Autodesk Inventor part; units mm, degrees
(part 4 of 4)
sketch "Sketch10" plane through (0, 0, 0) normal (0, 1, 0) x (1, 0, 0)
  circle A0 centre (29.25, 48.75) radius 2.8 construction
  circle A1 centre (29.25, 29.25) radius 2.8 construction
  circle A2 centre (29.25, 9.75) radius 2.8 construction
  circle A3 centre (29.25, -9.75) radius 2.8 construction
  circle A4 centre (29.25, -29.25) radius 2.8 construction
  circle A5 centre (29.25, -48.75) radius 2.8 construction
  circle A6 centre (9.75, 48.75) radius 2.8 construction
  circle A7 centre (-9.75, 48.75) radius 2.8 construction
  circle A8 centre (-29.25, 48.75) radius 2.8 construction
  circle A9 centre (29.25, 48.75) radius 2.8
  circle A10 centre (29.25, 29.25) radius 2.8
  circle A11 centre (29.25, 9.75) radius 2.8
  circle A12 centre (29.25, -9.75) radius 2.8
  circle A13 centre (29.25, -29.25) radius 2.8
  circle A14 centre (29.25, -48.75) radius 2.8
  circle A15 centre (9.75, 48.75) radius 2.8
  circle A16 centre (9.75, 29.25) radius 2.8
  circle A17 centre (9.75, 9.75) radius 2.8
  circle A18 centre (9.75, -9.75) radius 2.8
  circle A19 centre (9.75, -29.25) radius 2.8
  circle A20 centre (9.75, -48.75) radius 2.8
  circle A21 centre (-9.75, 48.75) radius 2.8
  circle A22 centre (-9.75, 29.25) radius 2.8
  circle A23 centre (-9.75, 9.75) radius 2.8
  circle A24 centre (-9.75, -9.75) radius 2.8
  circle A25 centre (-9.75, -29.25) radius 2.8
  circle A26 centre (-9.75, -48.75) radius 2.8
  circle A27 centre (-29.25, 48.75) radius 2.8
  circle A28 centre (-29.25, 29.25) radius 2.8
  circle A29 centre (-29.25, 9.75) radius 2.8
  circle A30 centre (-29.25, -9.75) radius 2.8
  circle A31 centre (-29.25, -29.25) radius 2.8
  circle A32 centre (-29.25, -48.75) radius 2.8
  point P0 (0, 0)
  dimension "d378" = 5.6
  dimension "d379" = 5.6
  dimension "d380" = 5.6
  dimension "d381" = 5.6
  dimension "d382" = 5.6
  dimension "d383" = 5.6
  dimension "d384" = 5.6
  dimension "d385" = 5.6
  dimension "d386" = 5.6
  dimension "d387" = 5.6
  dimension "d388" = 5.6
  dimension "d389" = 5.6
  dimension "d390" = 5.6
  dimension "d391" = 5.6
  dimension "d392" = 5.6
  dimension "d393" = 5.6
  dimension "d394" = 5.6
  dimension "d395" = 5.6
  dimension "d396" = 5.6
  dimension "d397" = 5.6
  dimension "d398" = 5.6
  dimension "d399" = 5.6
  dimension "d400" = 5.6
  dimension "d401" = 5.6
  constraints: 24 centre point, 6 coincident
  measures "d378" diameter of A9
  measures "d379" diameter of A10
  measures "d380" diameter of A11
  measures "d381" diameter of A12
  measures "d382" diameter of A13
  measures "d383" diameter of A14
  measures "d384" diameter of A15
  measures "d385" diameter of A16
  measures "d386" diameter of A17
  measures "d387" diameter of A18
  measures "d388" diameter of A19
  measures "d389" diameter of A20
  measures "d390" diameter of A21
  measures "d391" diameter of A22
  measures "d392" diameter of A23
  measures "d393" diameter of A24
  measures "d394" diameter of A25
  measures "d395" diameter of A26
  measures "d396" diameter of A27
  measures "d397" diameter of A28
  measures "d398" diameter of A29
  measures "d399" diameter of A30
  measures "d400" diameter of A31
  measures "d401" diameter of A32
sketch "Sketch11" plane through (0, 0, 0) normal (0, 1, 0) x (1, 0, 0)
  circle A0 centre (17.1945, 60.0191) radius 0.75 projected
  circle A1 centre (9.6945, 60.0191) radius 0.75 projected
  circle A2 centre (-2.3055, 60.0191) radius 0.75 projected
  circle A3 centre (-21.8055, 60.0191) radius 0.75 projected
  circle A4 centre (-29.3055, 60.0191) radius 0.75 projected
  circle A5 centre (29.3055, -60.0191) radius 0.75 projected
  circle A6 centre (21.8055, -60.0191) radius 0.75 projected
  circle A7 centre (9.8055, -60.0191) radius 0.75 projected
  circle A8 centre (2.3055, -60.0191) radius 0.75 projected
  circle A9 centre (-9.6945, -60.0191) radius 0.75 projected
  circle A10 centre (-17.1945, -60.0191) radius 0.75 projected
  line L0 (17.1945, 60.0191) -> (9.6945, 60.0191) construction
  circle A11 centre (-9.8055, 60.0191) radius 0.75 projected
  line L1 (-9.8055, 60.0191) -> (-2.3055, 60.0191) construction
  line L2 (-21.8055, 60.0191) -> (-29.3055, 60.0191) construction
  line L3 (-17.1945, -60.0191) -> (-9.6945, -60.0191) construction
  line L4 (2.3055, -60.0191) -> (9.8055, -60.0191) construction
  line L5 (29.3055, -60.0191) -> (21.8055, -60.0191) construction
  circle A12 centre (29.25, -48.75) radius 2.8 projected
  circle A13 centre (-29.25, 48.75) radius 2.8 projected
  line L6 (-29.25, 48.75) -> (-43.25, 48.75) construction
  line L7 (29.25, -48.75) -> (43.25, -48.75) construction
  circle A14 centre (43.25, -48.75) radius 1.25
  circle A15 centre (25.5555, -60.0191) radius 1.25
  circle A16 centre (6.0555, -60.0191) radius 1.25
  circle A17 centre (-13.4445, -60.0191) radius 1.25
  circle A18 centre (-25.5555, 60.0191) radius 1.25
  circle A19 centre (-6.0555, 60.0191) radius 1.25
  circle A20 centre (13.4445, 60.0191) radius 1.25
  circle A21 centre (-43.25, 48.75) radius 1.25
  point P0 (0, 0)
  dimension "d526" = 14
  dimension "d527" = 14
  dimension "d528" = 2.5
  dimension "d529" = 2.5
  dimension "d530" = 2.5
  dimension "d532" = 2.5
  dimension "d533" = 2.5
  dimension "d534" = 2.5
  dimension "d535" = 2.5
  dimension "d536" = 2.5
  constraints: 16 end point, 8 centre point, 8 horizontal, 6 midpoint, 2 coincident
  measures "d526" distance of L6.start L6.end
  measures "d527" distance of L7.start L7.end
  measures "d528" diameter of A14
  measures "d529" diameter of A15
  measures "d530" diameter of A16
  measures "d532" diameter of A17
  measures "d533" diameter of A18
  measures "d534" diameter of A19
  measures "d535" diameter of A20
  measures "d536" diameter of A21
extrude "Extrusion3" add sketch "Sketch7" along normal blind 6 contours A6 L10 L11 L9 | L9 L11 L10 A6 | L16 L15 A8 L14 | L14 A8 L15 L16 | A7 L29 L28 L27 | L27 L28 L29 A7 | L42 L41 A9 L40 | L40 A9 L41 L42 | L51 L50 A10 L49 | L49 A10 L50 L51 | A11 L155 L157 L156 | L156 L157 L155 A11 | A53 L185 L184 L183 | L183 L184 L185 A53 | L203 A54 L200 L189 | L189 L200 A54 L203 | L198 A55 L199 L190 | L190 L199 A55 L198 | L206 A56 L209 L191 | L191 L209 A56 L206 | A59 L204 L195 L192 | L192 L195 L204 A59 | L211 A60 L210 L205 | L205 L210 A60 L211 | A105 L335 L334 L333 | L333 L334 L335 A105 | L353 A106 L350 L339 | L339 L350 A106 L353 | L348 A107 L349 L340 | L340 L349 A107 L348 | L356 A108 L359 L341 | L341 L359 A108 L356 | A111 L354 L345 L342 | L342 L345 L354 A111 | L361 A112 L360 L355 | L355 L360 A112 L361 | A151 L485 L484 L483 | L483 L484 L485 A151 | L503 A152 L500 L489 | L489 L500 A152 L503 | L498 A153 L499 L490 | L490 L499 A153 L498 | L506 A154 L509 L491 | L491 L509 A154 L506 | A157 L504 L495 L492 | L492 L495 L504 A157 | L511 A158 L510 L505 | L505 L510 A158 L511 | A197 L635 L634 L633 | L633 L634 L635 A197 | L653 A198 L650 L639 | L639 L650 A198 L653 | L648 A199 L649 L640 | L640 L649 A199 L648 | L656 A200 L659 L641 | L641 L659 A200 L656 | A203 L654 L645 L642 | L642 L645 L654 A203 | L661 A204 L660 L655 | L655 L660 A204 L661 | L913 L917 L912 A269 | A269 L912 L917 L913 | A286 L780 L920 L779 | L779 L920 L780 A286 | A287 L784 L921 L787 | L787 L921 L784 A287 | A288 L791 L922 L792 | L792 L922 L791 A288 | L916 L796 A278 L795 | L795 A278 L796 L916 | L800 L803 A243 L799 | L799 A243 L803 L800 | L1063 L1067 L1062 A315 | A315 L1062 L1067 L1063 | A332 L930 L1070 L929 | L929 L1070 L930 A332 | A333 L934 L1071 L937 | L937 L1071 L934 A333 | A334 L941 L1072 L942 | L942 L1072 L941 A334 | L1066 L946 A324 L945 | L945 A324 L946 L1066 | L950 L953 A289 L949 | L949 A289 L953 L950 | L1213 L1217 L1212 A361 | A361 L1212 L1217 L1213 | A378 L1080 L1220 L1079 | L1079 L1220 L1080 A378 | A379 L1084 L1221 L1087 | L1087 L1221 L1084 A379 | A380 L1091 L1222 L1092 | L1092 L1222 L1091 A380 | L1216 L1096 A370 L1095 | L1095 A370 L1096 L1216 | L1100 L1103 A335 L1099 | L1099 A335 L1103 L1100
extrude "Extrusion4" add sketch "Sketch7" along normal blind 0.5 contours L3 A33 L65 A35 L76 L172 L77 A34 L67 A32 L4 A22 L6 A31 L10 A6 L9 A30 L5 A23 | A6 L10 L11 L9 | L14 A8 L15 L16 | L14 A29 L19 A20 L32 A37 L81 A45 L84 L118 L117 L173 L119 A44 L83 A36 L33 A21 L20 A28 L15 A8 | A45 L118 L84 | A19 L36 A39 L99 A47 L101 L123 L122 L174 L124 A46 L100 A38 L37 A18 L24 A27 L29 A7 L27 A26 L23 | A7 L29 L28 L27 | A47 L123 L101 | L40 A9 L41 L42 | L40 A25 L45 A17 L60 A41 L90 A49 L92 L115 L175 L127 A48 L91 A40 L61 A16 L46 A24 L41 A9 | A49 L126 L92 | L126 A49 L125 L175 L115 | L51 L50 A10 L49 | A10 L50 A13 L54 A14 L56 A43 L95 A50 L130 L176 L131 A51 L96 A42 L57 A15 L55 A12 L49 | L156 L157 L155 A11 | A11 L155 L177 L156 | L183 A53 L185 L188 | L183 L184 L185 A53 | L189 L200 A54 L203 | A54 L200 A63 L215 A68 L278 A93 L308 A96 L319 L321 L316 A95 L311 A94 L277 A65 L216 A64 L203 | L198 A55 L199 L190 | L198 A69 L218 A78 L286 A86 L264 A85 L263 L268 L270 L272 L269 A88 L266 A87 L283 A77 L221 A70 L199 A55 | A85 L268 L263 | L206 A56 L209 L191 | L206 A75 L231 A73 L232 A79 L239 A82 L245 L247 L240 A81 L237 A80 L233 A72 L228 A74 L209 A56 | A57 L223 A66 L282 A89 L296 A92 L291 L301 L299 L297 L298 A91 L292 A90 L279 A67 L224 A58 L204 A59 L192 | A59 L204 L195 L192 | A92 L301 L291 | L205 L210 A60 L211 | A60 L210 A62 L229 A76 L288 A97 L324 A84 L262 L258 L253 L256 A83 L327 A98 L287 A71 L226 A61 L211 | A84 L261 L262 | L261 A84 L257 L253 L258 | L333 A105 L335 L338 | L333 L334 L335 A105 | L339 L350 A106 L353 | A106 L350 A115 L365 A120 L428 A145 L458 A148 L469 L471 L466 A147 L461 A146 L427 A117 L366 A116 L353 | L348 A107 L349 L340 | L348 A121 L368 A130 L436 A138 L414 A137 L413 L418 L420 L422 L419 A140 L416 A139 L433 A129 L371 A122 L349 A107 | A137 L418 L413 | L356 A108 L359 L341 | L356 A127 L381 A125 L382 A131 L389 A134 L395 L397 L390 A133 L387 A132 L383 A124 L378 A126 L359 A108 | A109 L373 A118 L432 A141 L446 A144 L441 L451 L449 L447 L448 A143 L442 A142 L429 A119 L374 A110 L354 A111 L342 | A111 L354 L345 L342 | A144 L451 L441 | L355 L360 A112 L361 | A112 L360 A114 L379 A128 L438 A149 L474 A136 L412 L408 L403 L406 A135 L477 A150 L437 A123 L376 A113 L361 | A136 L411 L412 | L411 A136 L407 L403 L408 | L483 A151 L485 L488 | L483 L484 L485 A151 | L489 L500 A152 L503 | A152 L500 A161 L515 A166 L578 A191 L608 A194 L619 L621 L616 A193 L611 A192 L577 A163 L516 A162 L503 | L498 A153 L499 L490 | L498 A167 L518 A176 L586 A184 L564 A183 L563 L568 L570 L572 L569 A186 L566 A185 L583 A175 L521 A168 L499 A153 | A183 L568 L563 | L506 A154 L509 L491 | L506 A173 L531 A171 L532 A177 L539 A180 L545 L547 L540 A179 L537 A178 L533 A170 L528 A172 L509 A154 | A155 L523 A164 L582 A187 L596 A190 L591 L601 L599 L597 L598 A189 L592 A188 L579 A165 L524 A156 L504 A157 L492 | A157 L504 L495 L492 | A190 L601 L591 | L505 L510 A158 L511 | A158 L510 A160 L529 A174 L588 A195 L624 A182 L562 L558 L553 L556 A181 L627 A196 L587 A169 L526 A159 L511 | A182 L561 L562 | L561 A182 L557 L553 L558 | L633 A197 L635 L638 | L633 L634 L635 A197 | L639 L650 A198 L653 | A198 L650 A207 L665 A212 L728 A237 L758 A240 L769 L771 L766 A239 L761 A238 L727 A209 L666 A208 L653 | L648 A199 L649 L640 | L648 A213 L668 A222 L736 A230 L714 A229 L713 L718 L720 L722 L719 A232 L716 A231 L733 A221 L671 A214 L649 A199 | A229 L718 L713 | L656 A200 L659 L641 | L656 A219 L681 A217 L682 A223 L689 A226 L695 L697 L690 A225 L687 A224 L683 A216 L678 A218 L659 A200 | A201 L673 A210 L732 A233 L746 A236 L741 L751 L749 L747 L748 A235 L742 A234 L729 A211 L674 A202 L654 A203 L642 | A203 L654 L645 L642 | A236 L751 L741 | L655 L660 A204 L661 | A204 L660 A206 L679 A220 L738 A241 L774 A228 L712 L708 L703 L706 A227 L777 A242 L737 A215 L676 A205 L661 | A228 L711 L712 | L711 A228 L707 L703 L708 | L778 A276 L813 A261 L898 A268 L900 L908 L905 L903 L904 A267 L899 A262 L814 A277 L821 A273 L912 A269 L913 A272 | A269 L912 L917 L913 | A268 L908 L900 | L779 A286 L780 A283 L789 A245 L836 A254 L846 A255 L845 L851 L854 L859 A256 L849 A253 L837 A279 L918 A280 | L779 L920 L780 A286 | L851 L850 A255 L858 L854 | A255 L850 L845 | A281 L809 A258 L862 A259 L864 L867 L872 L871 L870 A260 L863 A257 L812 A282 L806 A271 L784 A287 L787 A270 L783 | A287 L784 L921 L787 | A259 L867 L864 | A248 L822 A249 L826 A251 L834 L833 L830 A252 L828 A250 L823 A246 L835 A244 L791 A288 L792 A247 L790 | A288 L791 L922 L792 | L795 A278 L796 L916 | L795 A285 L808 A275 L816 A264 L877 A266 L889 L894 L888 A265 L879 A263 L817 A274 L909 A284 L796 A278 | L799 A243 L803 L800 | L799 L802 L803 A243 | L928 A322 L963 A307 L1048 A314 L1050 L1058 L1055 L1053 L1054 A313 L1049 A308 L964 A323 L971 A319 L1062 A315 L1063 A318 | A315 L1062 L1067 L1063 | A314 L1058 L1050 | L929 A332 L930 A329 L939 A291 L986 A300 L996 A301 L995 L1001 L1004 L1009 A302 L999 A299 L987 A325 L1068 A326 | L929 L1070 L930 A332 | L1001 L1000 A301 L1008 L1004 | A301 L1000 L995 | A327 L959 A304 L1012 A305 L1014 L1017 L1022 L1021 L1020 A306 L1013 A303 L962 A328 L956 A317 L934 A333 L937 A316 L933 | A333 L934 L1071 L937 | A305 L1017 L1014 | A294 L972 A295 L976 A297 L984 L983 L980 A298 L978 A296 L973 A292 L985 A290 L941 A334 L942 A293 L940 | A334 L941 L1072 L942 | L945 A324 L946 L1066 | L945 A331 L958 A321 L966 A310 L1027 A312 L1039 L1044 L1038 A311 L1029 A309 L967 A320 L1059 A330 L946 A324 | L949 A289 L953 L950 | L949 L952 L953 A289 | L1078 A368 L1113 A353 L1198 A360 L1200 L1208 L1205 L1203 L1204 A359 L1199 A354 L1114 A369 L1121 A365 L1212 A361 L1213 A364 | A361 L1212 L1217 L1213 | A360 L1208 L1200 | L1079 A378 L1080 A375 L1089 A337 L1136 A346 L1146 A347 L1145 L1151 L1154 L1159 A348 L1149 A345 L1137 A371 L1218 A372 | L1079 L1220 L1080 A378 | L1151 L1150 A347 L1158 L1154 | A347 L1150 L1145 | A373 L1109 A350 L1162 A351 L1164 L1167 L1172 L1171 L1170 A352 L1163 A349 L1112 A374 L1106 A363 L1084 A379 L1087 A362 L1083 | A379 L1084 L1221 L1087 | A351 L1167 L1164 | A340 L1122 A341 L1126 A343 L1134 L1133 L1130 A344 L1128 A342 L1123 A338 L1135 A336 L1091 A380 L1092 A339 L1090 | A380 L1091 L1222 L1092 | L1095 A370 L1096 L1216 | L1095 A377 L1108 A367 L1116 A356 L1177 A358 L1189 L1194 L1188 A357 L1179 A355 L1117 A366 L1209 A376 L1096 A370 | L1099 A335 L1103 L1100 | L1099 L1102 L1103 A335 picked at (41.2772, -59.7704) picked at (39.0702, -55.2707) picked at (37.2772, -59.7707) picked at (35.0702, -55.2707) picked at (33.2772, -59.7707) picked at (29.3405, -59.7709) picked at (29.1595, 59.7709) picked at (17.1662, 59.7704) picked at (21.2228, 59.7707) picked at (25.2228, 59.7707) picked at (19.4864, 55.2707) picked at (23.4864, 55.2707) picked at (9.6595, 59.7709) picked at (-2.3338, 59.7704) picked at (1.7228, 59.7707) picked at (5.7228, 59.7707) picked at (-0.0136, 55.2707) picked at (3.9864, 55.2707) picked at (-9.8405, 59.7709) picked at (-21.8338, 59.7704) picked at (-17.7772, 59.7707) picked at (-13.8338, 59.7707) picked at (-19.5136, 55.2707) picked at (-15.5702, 55.2707) picked at (-29.3405, 59.7709) picked at (-41.3338, 59.7704) picked at (-37.3338, 59.7707) picked at (-33.3338, 59.7707) picked at (-39.0702, 55.2707) picked at (-35.0702, 55.2707) picked at (19.5702, -55.2707) picked at (15.5702, -55.2707) picked at (17.8338, -59.7707) picked at (13.8338, -59.7707) picked at (21.7772, -59.7704) picked at (9.8405, -59.7709) picked at (0.0702, -55.2707) picked at (-3.9298, -55.2707) picked at (-1.6662, -59.7707) picked at (-5.6662, -59.7707) picked at (2.2772, -59.7704) picked at (-9.6595, -59.7709) picked at (-19.4298, -55.2707) picked at (-23.4298, -55.2707) picked at (-21.1662, -59.7707) picked at (-25.1662, -59.7707) picked at (-17.2228, -59.7704) picked at (-29.1595, -59.7709)
extrude "Extrusion5" add sketch "Sketch10" along normal blind 6
extrude "Extrusion6" add sketch "Sketch7" along normal blind 4 contours L163 L74 L75 L73 L162 L172 | L164 L135 L134 L136 L165 L173 | L166 L139 L138 L140 L167 L174 | L175 L168 L142 L141 L143 L169 | L176 L147 L145 L144 L146 L148 | L177 L160 L153 L152 L154 L161 | L179 L188 L181 L182 L180 L178 | L322 L315 L314 L318 L317 L321 | L272 L273 L276 L275 L274 L271 | L248 L249 L246 L242 L241 L247 | L304 L305 L303 L307 L306 L297 | L253 L255 L254 L250 L251 L252 | L329 L338 L331 L332 L330 L328 | L472 L465 L464 L468 L467 L471 | L422 L423 L426 L425 L424 L421 | L398 L399 L396 L392 L391 L397 | L454 L455 L453 L457 L456 L447 | L403 L405 L404 L400 L401 L402 | L479 L488 L481 L482 L480 L478 | L622 L615 L614 L618 L617 L621 | L572 L573 L576 L575 L574 L571 | L548 L549 L546 L542 L541 L547 | L604 L605 L603 L607 L606 L597 | L553 L555 L554 L550 L551 L552 | L629 L638 L631 L632 L630 L628 | L772 L765 L764 L768 L767 L771 | L722 L723 L726 L725 L724 L721 | L698 L699 L696 L692 L691 L697 | L754 L755 L753 L757 L756 L747 | L703 L705 L704 L700 L701 L702 | L885 L884 L886 L883 L882 L903 | L854 L855 L857 L856 L861 L860 | L875 L874 L873 L868 L869 L871 | L840 L842 L843 L844 L841 L833 | L896 L897 L887 L892 L893 L894 | L926 L927 L923 L925 L924 L802 | L1035 L1034 L1036 L1033 L1032 L1053 | L1004 L1005 L1007 L1006 L1011 L1010 | L1025 L1024 L1023 L1018 L1019 L1021 | L990 L992 L993 L994 L991 L983 | L1046 L1047 L1037 L1042 L1043 L1044 | L1076 L1077 L1073 L1075 L1074 L952 | L1185 L1184 L1186 L1183 L1182 L1203 | L1154 L1155 L1157 L1156 L1161 L1160 | L1175 L1174 L1173 L1168 L1169 L1171 | L1140 L1142 L1143 L1144 L1141 L1133 | L1196 L1197 L1187 L1192 L1193 L1194 | L1226 L1227 L1223 L1225 L1224 L1102
extrude "Extrusion7" add sketch "Sketch11" along normal blind 6 contours A14 | A15 | A16 | A17 | A18 | A19 | A20 | A21
extrude "Extrusion8" cut sketch "Sketch3" against normal blind 1 contours L41 L38 L44 L30
fillet "Fillet1" radius 2 12 edges at (53.8, -8, 0) (50.3, -8, 66.5) (46.8, -8, 67.75) (0, -8, 69) (-46.8, -8, 67.75) (-50.3, -8, 66.5) (-53.8, -8, 0) (-50.3, -8, -66.5) (-46.8, -8, -67.75) (0, -8, -69) (46.8, -8, -67.75) (50.3, -8, -66.5)
body "Solid1"
